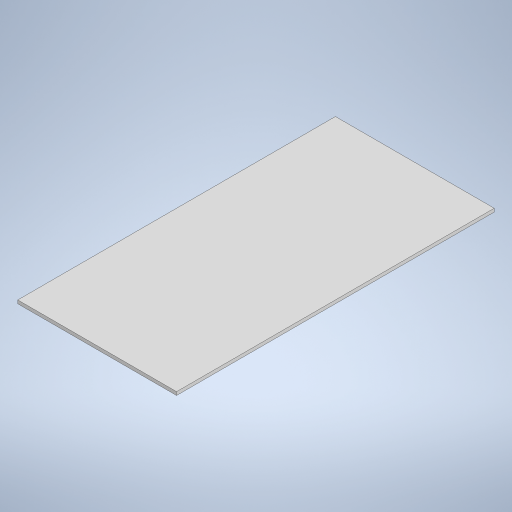
# Autodesk Inventor part: OdorMachineShelf
Saved by Autodesk Inventor 2023 (Build 270158000, 158)
## iProperties
Created: 2023-06-14
Part Number: OdorMachineShelf
Material: Generic
Document SubType Name: Modeling
Designer: User
Density: 1 g/cm^3
Appearance: Default
Author: User
Autodesk Inventor part; units mm, degrees
ref_plane "YZ Plane" through (0, 0, 0) normal (1, 0, 0) x (0, 1, 0)
ref_plane "XZ Plane" through (0, 0, 0) normal (0, 1, 0) x (-1, 0, 0)
ref_plane "XY Plane" through (0, 0, 0) normal (0, 0, 1) x (1, 0, 0)
sketch "Sketch1" plane through (0, 0, 0) normal (0, 1, 0) x (-1, 0, 0)
  line L0 (-152.4, 304.8) -> (152.4, 304.8)
  line L1 (152.4, 304.8) -> (152.4, -304.8)
  line L2 (152.4, -304.8) -> (-152.4, -304.8)
  line L3 (-152.4, -304.8) -> (-152.4, 304.8)
  line L4 (-152.4, 304.8) -> (152.4, -304.8) construction
  line L5 (152.4, 304.8) -> (-152.4, -304.8) construction
  point P0 (0, 0)
  dimension "d0" = 609.6
  dimension "d1" = 304.8
  constraints: 12 end point, 2 midpoint, 2 parallel, 1 horizontal, 1 perpendicular
  measures "d0" distance of L0.end L1.end
  measures "d1" distance of L1.end L2.end
extrude "Extrusion1" add sketch "Sketch1" along normal blind 6.35
body "Solid1"
